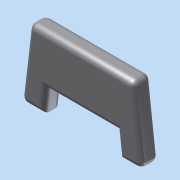
# Autodesk Inventor part: RUCBase
Saved by Autodesk Inventor 2011 SP1 (Build 150282100, 282)
## iProperties
Created: 2011-08-15
Part Number: RUCBase
Document SubType Name: Modeling
Designer: dgitz
Density: 1 g/cm^3
Author: dgitz
Autodesk Inventor part; units mm, degrees
ref_plane "YZ Plane" through (0, 0, 0) normal (1, 0, 0) x (0, 1, 0)
ref_plane "XZ Plane" through (0, 0, 0) normal (0, 1, 0) x (-1, 0, 0)
ref_plane "XY Plane" through (0, 0, 0) normal (0, 0, 1) x (1, 0, 0)
sketch "Sketch1" plane through (0, 0, 0) normal (0, 0, 1) x (1, 0, 0)
  line L0 (-53.184, 74.7028) -> (-72.234, -84.0472)
  line L1 (-72.234, -84.0472) -> (-21.434, -84.0472)
  line L2 (-21.434, -84.0472) -> (-15.338, -33.2472)
  line L3 (-15.338, -33.2472) -> (137.57, -33.2472)
  line L4 (137.57, -33.2472) -> (143.666, -84.0472)
  line L5 (143.666, -84.0472) -> (194.466, -84.0472)
  line L6 (194.466, -84.0472) -> (175.416, 74.7028)
  line L7 (175.416, 74.7028) -> (-53.184, 74.7028)
  point P0 (0, 0)
  dimension "d0" = 50.8
  dimension "d5" = 266.7
  dimension "d6" = 50.8
  dimension "d7" = 158.75
  dimension "d8" = 228.6
  dimension "d12" = 96.843
  dimension "d13" = 96.843
  constraints: 16 end point, 3 equal length, 3 horizontal, 3 parallel
  measures "d0" distance of L1.end L0.end
  measures "d5" distance of L5.end L0.end
  measures "d6" distance between parallel lines of L3 L1
  measures "d7" distance between parallel lines of L7 L1
  measures "d8" distance of L6.end L0.start
  measures "d12" angle of L0 L7
  measures "d13" angle of L6 L7
extrude "Extrusion1" add sketch "Sketch1" along normal blind 38.1
fillet "Fillet1" radius 12.7 20 edges at (61.116, 74.7028, 38.1) (-62.709, -4.6722, 38.1) (-46.834, -84.0472, 38.1) (-18.386, -58.6472, 38.1) (61.116, -33.2472, 38.1) (140.618, -58.6472, 38.1) (169.066, -84.0472, 38.1) (184.941, -4.6722, 38.1) (61.116, 74.7028, 0) (-62.709, -4.6722, 0) (-46.834, -84.0472, 0) (-18.386, -58.6472, 0) (61.116, -33.2472, 0) (140.618, -58.6472, 0) (169.066, -84.0472, 0) (184.941, -4.6722, 0) (175.416, 74.7028, 19.05) (194.466, -84.0472, 19.05) (-53.184, 74.7028, 19.05) (-72.234, -84.0472, 19.05)
body "Solid1"
